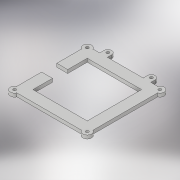
# Autodesk Inventor part: trellisCaptiveTop
Saved by Autodesk Inventor 2017 (Build 210142000, 142)
## iProperties
Created: 2017-05-22
Part Number: trellisCaptiveTop
Material: Generic
Document SubType Name: Modeling
Designer: Dominic Gaiero
Density: 1 g/cm^3
Appearance: Default
Author: Dominic Gaiero
Autodesk Inventor part; units mm, degrees
ref_plane "YZ Plane" through (0, 0, 0) normal (1, 0, 0) x (0, 1, 0)
ref_plane "XZ Plane" through (0, 0, 0) normal (0, 1, 0) x (-1, 0, 0)
ref_plane "XY Plane" through (0, 0, 0) normal (0, 0, 1) x (1, 0, 0)
sketch "Sketch1" plane through (0, 0, 0) normal (0, 1, 0) x (-1, 0, 0)
  line L0 (405.5305, 409.815) -> (465.5305, 409.815) construction
  line L1 (405.5305, 379.815) -> (405.5305, 409.815) construction
  line L2 (460.5305, 404.815) -> (410.5305, 404.815)
  line L3 (410.5305, 404.815) -> (410.5305, 379.815)
  line L4 (460.5305, 386.815) -> (470.5305, 386.815)
  line L5 (470.5305, 414.815) -> (465.2753, 414.815)
  line L6 (400.5305, 414.815) -> (400.5305, 409.5598) construction
  line L7 (465.5305, 409.815) -> (465.5305, 386.815) construction
  line L8 (460.5305, 386.815) -> (460.5305, 404.815)
  line L9 (470.5305, 386.815) -> (470.5305, 409.5598)
  line L10 (405.5305, 409.815) -> (400.5305, 414.815) construction
  line L11 (400.5305, 379.815) -> (470.5305, 379.815) construction
  line L12 (465.5305, 409.815) -> (470.5305, 414.815) construction
  arc A0 (405.7856, 414.815) -> (400.5305, 409.5598) centre (402.1112, 413.2342) ccw
  arc A1 (404.9397, 410.4058) -> (405.7856, 414.815) centre (402.1112, 413.2342) ccw construction
  line L13 (400.5305, 409.5598) -> (400.5305, 379.815)
  arc A2 (400.5305, 409.5598) -> (404.9397, 410.4058) centre (402.1112, 413.2342) ccw construction
  line L14 (405.7856, 414.815) -> (400.5305, 414.815) construction
  circle A3 centre (402.1112, 413.2342) radius 1.3
  line L15 (435.5305, 414.815) -> (435.5305, 379.815) construction
  arc A4 (465.2753, 414.815) -> (470.5305, 409.5598) centre (468.9497, 413.2342) ccw construction
  arc A5 (470.5305, 409.5598) -> (465.2753, 414.815) centre (468.9497, 413.2342) ccw
  line L16 (470.5305, 409.5598) -> (470.5305, 414.815) construction
  line L17 (465.2753, 414.815) -> (405.7856, 414.815)
  circle A6 centre (468.9497, 413.2342) radius 1.3
  line L18 (460.5305, 372.815) -> (460.5305, 354.815)
  line L19 (465.5305, 349.815) -> (465.5305, 372.815) construction
  line L20 (460.5305, 372.815) -> (470.5305, 372.815)
  line L21 (470.5305, 372.815) -> (470.5305, 350.0701)
  arc A7 (470.5305, 350.0701) -> (465.2753, 344.815) centre (468.9497, 346.3957) ccw construction
  line L22 (470.5305, 344.815) -> (465.2753, 344.815) construction
  line L23 (465.5305, 349.815) -> (470.5305, 344.815) construction
  line L24 (470.5305, 350.0701) -> (470.5305, 344.815) construction
  arc A8 (465.2753, 344.815) -> (470.5305, 350.0701) centre (468.9497, 346.3957) ccw
  circle A9 centre (468.9497, 346.3957) radius 1.3
  line L25 (400.5305, 344.815) -> (400.5305, 350.0701) construction
  circle A10 centre (402.1112, 346.3957) radius 1.3
  line L26 (405.5305, 349.815) -> (400.5305, 344.815) construction
  line L27 (405.7856, 344.815) -> (400.5305, 344.815) construction
  arc A11 (400.5305, 350.0701) -> (405.7856, 344.815) centre (402.1112, 346.3957) ccw
  line L28 (435.5305, 344.815) -> (435.5305, 379.815) construction
  line L29 (405.5305, 349.815) -> (465.5305, 349.815) construction
  line L30 (460.5305, 354.815) -> (410.5305, 354.815)
  arc A12 (405.7856, 344.815) -> (404.9397, 349.2242) centre (402.1112, 346.3957) ccw construction
  line L31 (410.5305, 354.815) -> (410.5305, 379.815)
  line L32 (405.5305, 379.815) -> (405.5305, 349.815)
  line L33 (400.5305, 350.0701) -> (400.5305, 379.815)
  arc A13 (404.9397, 349.2242) -> (400.5305, 350.0701) centre (402.1112, 346.3957) ccw construction
  circle A14 centre (415.5305, 340.824) radius 1.3
  arc A15 (412.0305, 340.824) -> (419.0305, 340.824) centre (415.5305, 340.824) ccw
  line L34 (412.0305, 340.824) -> (412.0305, 344.815)
  line L35 (419.0305, 340.824) -> (419.0305, 344.815)
  line L36 (452.0305, 340.824) -> (452.0305, 344.815)
  circle A16 centre (455.5305, 340.824) radius 1.3
  arc A17 (452.0305, 340.824) -> (459.0305, 340.824) centre (455.5305, 340.824) ccw
  line L37 (459.0305, 340.824) -> (459.0305, 344.815)
  line L38 (412.0305, 344.815) -> (405.7856, 344.815)
  line L39 (465.2753, 344.815) -> (459.0305, 344.815)
  line L40 (452.0305, 344.815) -> (419.0305, 344.815)
  point P0 (0, 0)
  point P1 (403.0305, 412.315)
  point P2 (468.0305, 412.315)
  point P3 (468.0305, 347.315)
  point P4 (403.0305, 347.315)
  dimension "d0" = 23
  dimension "d1" = 5
  dimension "d2" = 8
  dimension "d3" = 2.6
  dimension "d4" = 8
  dimension "d5" = 2.6
  dimension "d6" = 2.6
  dimension "d7" = 20
  dimension "d8" = 35
  dimension "d9" = 7
  constraints: 82 end point, 27 symmetric about line, 24 point on circle, 18 centre point, 12 perpendicular, 10 point on line, 6 parallel, 5 midpoint, 4 coincident, 2 horizontal, 2 tangent, 1 vertical, 9 other
  measures "d0" distance between parallel lines of L0 L4
  measures "d1" distance between parallel lines of L0 L5
  measures "d2" diameter of A0
  measures "d3" diameter of A3
  measures "d4" diameter of A4
  measures "d5" diameter of A6
  measures "d6" diameter of A14
  measures "d7" distance from line of L28 A14.centre
  measures "d8" distance between parallel lines of L21 L28
  measures "d9" diameter of A15
extrude "Extrusion1" add sketch "Sketch1" along normal blind 3.175
body "Solid1"
